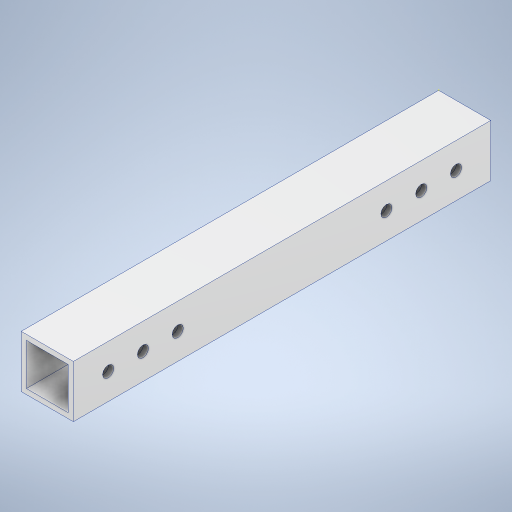
# Autodesk Inventor part: 射出_角柱12
Saved by Autodesk Inventor 2023 (Build 270158000, 158)
## iProperties
Created: 2022-04-20
Part Number: 射出_角柱12
Material: アルミニウム 6061
Document SubType Name: Modeling
Designer: yuta
Density: 2.7 g/cm^3
Appearance: アルミニウム - フラット
Author: yuta
Autodesk Inventor part; units mm, degrees
ref_plane "YZ Plane" through (0, 0, 0) normal (1, 0, 0) x (0, 1, 0)
ref_plane "XZ Plane" through (0, 0, 0) normal (0, 1, 0) x (-1, 0, 0)
ref_plane "XY Plane" through (0, 0, 0) normal (0, 0, 1) x (1, 0, 0)
sketch "スケッチ1" plane through (0, 0, 0) normal (0, 0, 1) x (1, 0, 0)
  line L0 (0, 0) -> (15, 0)
  line L1 (15, 0) -> (15, 15)
  line L2 (15, 15) -> (0, 15)
  line L3 (0, 15) -> (0, 0)
  dimension "d0" = 15
  dimension "d1" = 15
  constraints: 8 end point, 2 parallel, 1 horizontal, 1 perpendicular
  measures "d0" distance of L2.end L1.end
  measures "d1" distance of L1.end L0.end
extrude "押し出し1" add sketch "スケッチ1" along normal blind 120
sketch "スケッチ2" plane through (0, 15, 0) normal (0, 1, 0) x (1, 0, 0)
  point P0 (0, 0)
sketch "スケッチ3" plane through (15, 0, 0) normal (1, 0, 0) x (0, 0, -1)
  line L0 (-120, 0) -> (-120, 15) projected
  line L1 (0, 0) -> (-120, 0) projected
  line L2 (0, 0) -> (0, 15) projected
  point P0 (-110, 7.5)
  point P1 (-100, 7.5)
  point P2 (-90, 7.5)
  point P3 (-30, 7.5)
  point P4 (-20, 7.5)
  point P5 (-10, 7.5)
  dimension "d4" = 10
  dimension "d5" = 7.5
  dimension "d6" = 10
  dimension "d7" = 10
  dimension "d8" = 7.5
  dimension "d9" = 7.5
  dimension "d10" = 7.5
  dimension "d11" = 30
  dimension "d12" = 20
  dimension "d13" = 7.5
  dimension "d14" = 7.5
  dimension "d15" = 10
  measures "d4" distance from line of L0 point (-110, 7.5)
  measures "d5" distance from line of L1 point (-110, 7.5)
  measures "d6" distance of point (-110, 7.5) point (-100, 7.5)
  measures "d7" distance of point (-100, 7.5) point (-90, 7.5)
  measures "d8" distance from line of L1 point (-100, 7.5)
  measures "d9" distance from line of L1 point (-90, 7.5)
  measures "d10" distance from line of L1 point (-30, 7.5)
  measures "d11" distance from line of L2 point (-30, 7.5)
  measures "d12" distance from line of L2 point (-20, 7.5)
  measures "d13" distance from line of L1 point (-10, 7.5)
  measures "d14" distance from line of L1 point (-20, 7.5)
  measures "d15" distance from line of L2 point (-10, 7.5)
hole "穴1" at (15, 7.5, 110) at (15, 7.5, 100) at (15, 7.5, 90) at (15, 7.5, 30) at (15, 7.5, 20) at (15, 7.5, 10) direction (-1, 0, 0) diameter 3.2 end through all
sketch "スケッチ4" plane through (0, 0, 120) normal (0, 0, 1) x (1, 0, 0)
  line L0 (1.5, 13.5) -> (13.5, 13.5)
  line L1 (13.5, 13.5) -> (13.5, 1.5)
  line L2 (13.5, 1.5) -> (1.5, 1.5)
  line L3 (1.5, 1.5) -> (1.5, 13.5)
  line L4 (15, 15) -> (0, 15) projected
  line L5 (0, 15) -> (0, 0) projected
  dimension "d23" = 12
  dimension "d24" = 12
  dimension "d25" = 1.5
  dimension "d26" = 1.5
  constraints: 8 end point, 2 parallel, 1 horizontal, 1 perpendicular
  measures "d23" distance of L1.end L2.end
  measures "d24" distance of L0.end L1.end
  measures "d25" distance between parallel lines of L4 L0
  measures "d26" distance between parallel lines of L5 L3
extrude "押し出し2" cut sketch "スケッチ4" against normal blind 600
